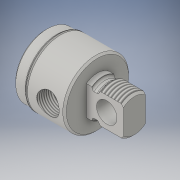
# Autodesk Inventor part: 09P0Y000_rear_head
Saved by Autodesk Inventor 2016 SP1 (Build 200210100, 210)
## iProperties
Category: PARTsolutions
Company: BIMBA
Created: 2017-03-09
Part Number: 09P0Y000_rear_head
Material: Generic
Catalog Web Link: www.cadenas.de
Description: Rear Head-Original Line - Standard Air Cylinders
Vendor: BIMBA
Document SubType Name: Standard Catalog Part
Designer: 589013
Manufacturer: BIMBA
Mass: 12.8763 g
Surface Area: 50.2035 cm^2
Volume: 12.8763 cm^3
Density: 1 g/cm^3
Appearance: PSOLRGB-211-211-211
PSOL_IDENT_0: {$CADENAS_DATA\23d-libs\bimba\bimba\bimba_imperial\bimba_full_line\original_line_cylinders\standard_
PSOL_IDENT_1: air_cylinders\rear_head.prj},231 {VTYP=3D},{NB=09P0Y000_rear_head},{LINA=09P0Y000_rear_head},{NN=Rea
PSOL_IDENT_2: r Head},{DATE=09.11.2016 07:55:11},{GEOMDATE=30.06.2014 06:34:00},{VERSION=},{LINEID=60},{LINESUBID=
PSOL_IDENT_3: -1},{WBVAR=MNT,ACTING,DER,Q,T1,T2,T3,T4,TRIM,Y,K,MB,CUSH,FBON}  {NB=09P0Y000_rear_head},{LINA=09P0Y0
PSOL_IDENT_4: 00_rear_head},{KT=DUMMY},{PN=09P0Y000},{BORE=1.06250},{BOREPN=09},{MNT=P},{MNTALG='' , 'Front Nose'
PSOL_IDENT_5: , 'P' , 'Rear Pivot' , 'S' , 'Built-in Valve S' , 'LS' , 'Built-in Valve LS' , 'DX' , 'Double End' ,
PSOL_IDENT_6: 'BR' , 'Rear Block' , 'BRT' , 'Rear Trunnion' , 'A' , 'Adjustable Stroke' , 'M' , 'Manual Valve'},{
PSOL_IDENT_7: ACTING=},{ACTINGALG= '' , 'Single Acting' , 'R' , 'Reverse/Double Acting' },{DER=},{DERALG= '' , 'St
PSOL_IDENT_8: andard' },{Q=},{T1=},{T2=},{T3=},{T4=},{TRIM=0},{Y=Y},{K=},{KALG= '', 'without K', 'K', 'with K' },{
PSOL_IDENT_9: MB=0},{A1=1.5000},{A1N=0.6250},{A1P=1.5000},{A1B=1.1250},{A1S=1.1250},{A2=0.25},{A2N=0.2500},{A3=0.0
PSOL_IDENT_10: 300},{D1=1.1110},{D1N=1.1155},{D1P=1.1110},{D1B=1.1410},{D2=1.0715},{C1=0.0300},{C2=0.0300},{NDM=0.4
PSOL_IDENT_11: 050},{TAB=NPT},{NDMDP=0.2730},{D3=0.3440},{A4=0.1880},{A5=0.8700},{D4=0.0000},{A6=0.0000},{A7=0.6250
PSOL_IDENT_12: },{A8=0.0000},{D5=0.0000},{D6=0.3750},{A9=0.7500},{NDM2=0.6250},{TAB2=UNF},{C11=0.0300},{C22=0.0000}
PSOL_IDENT_13: ,{C33=0.0000},{C44=0.0300},{A10=0.3725},{A11=0.0000},{NDM3=0.4050},{NDM3N=0.4050},{NDM3B=0.4050},{TA
PSOL_IDENT_14: B3=NPT},{TAB3N=NPT},{TAB3B=NPT},{A12=0.594},{A12N=0.5940},{A12B=0.6880},{A13=1.2190},{D7=0.2520},{D8=
PSOL_IDENT_15: 0.6225},{A14=0.0940},{A15=0.0855},{D9=0.5385},{R1=0.0350},{X1=0.0000},{X2=0.0000},{CX=0.0000},{CC=0.
PSOL_IDENT_16: 0000},{CON=1},{S1=1.2500},{DB=0.2500},{X1B=0.0000},{X2B=0.0000},{A8B=0.1250},{A9B=0.8800},{MODEL=1},
PSOL_IDENT_17: {NDM4=0.1900},{TAB4=UNF},{NDM4DP=0.3120},{BC=1.2500},{B1=0.7500},{B2=0.3800},{B3=0.5000},{ON=0},{ON2=
PSOL_IDENT_18: 1},{G1=0.3440},{G2=0.8120},{G3=0.6250},{G4=0.6245},{GD=0.2520},{G5=0.7180},{G6=0.3725},{RON=0},{H1=0
PSOL_IDENT_19: .0000},{H2=1.1300},{H3=0.1250},{H4=0.0000},{H5=0.0000},{H6=0.0000},{F=0.5000},{PNUT=0.9690},{CUSH=0}
PSOL_IDENT_20: ,{CC11=0.278},{CC111=0.2775},{CC22=0.4045},{CC33=0.2450},{CC44=0.5350},{CC55=0.7000},{CD1=0.2050},{C
PSOL_IDENT_21: D2=0.1360},{CD3=0.0775},{CNDM3=0.1900},{CTAB3=UNS},{OLEN=1.2190},{OD=0.3455},{STDIS=0.2500},{STDIS1=
PSOL_IDENT_22: 0.2500},{BUSHCON=D-3543},{BUSHL=0.3700},{FBON=0},{LCD=0.0000}
NN: Rear Head
NT: Original Line - Standard Air Cylinders
NB: 09P0Y000_rear_head
NBSYN: $PN._rear_head
LINA: 09P0Y000_rear_head
PN: 09P0Y000
BORE: 1.06250
BOREPN: 09
MNT: Rear Pivot
MNTALG: '' , 'Front Nose' , 'P' , 'Rear Pivot' , 'S' , 'Built-in Valve S' , 'LS' , 'Built-in Valve LS' , 'DX' , 'Double End' , 'BR' , 'Rear Block' , 'BRT' , 'Rear Trunnion' , 'A' , 'Adjustable Stroke' , 'M' , 'Manual Valve'
ACTING: Single Acting
DER: Standard
Q: Without Side Ported Rear Head
T1: without T1
T2: without T2
T3: without T3
T4: without T4
TRIM: 0
Y: with Pivot Bushing
K: without K
MB: 0
A1N: 0.6250
A1P: 1.5000
A1B: 1.1250
A1S: 1.1250
A2N: 0.2500
A3: 0.0300
D1N: 1.1155
D1P: 1.1110
D1B: 1.1410
D2: 1.0715
C1: 0.0300
C2: 0.0300
TAB: NPT
NDMDP: 0.2730
D3: 0.3440
A4: 0.1880
A5: 0.8700
D4: 0.0000
A6: 0.0000
A7: 0.6250
A8: 0.0000
D5: 0.0000
D6: 0.3750
A9: 0.7500
NDM2: 0.6250
TAB2: UNF
C11: 0.0300
C22: 0.0000
C33: 0.0000
C44: 0.0300
A10: 0.3725
A11: 0.0000
NDM3N: 0.4050
NDM3B: 0.4050
TAB3N: NPT
TAB3B: NPT
A12N: 0.5940
A12B: 0.6880
A13: 1.2190
D7: 0.2520
D8: 0.6225
A14: 0.0940
A15: 0.0855
D9: 0.5385
R1: 0.0350
X1: 0.0000
X2: 0.0000
CX: 0.0000
CC: 0.0000
S1: 1.2500
DB: 0.2500
X1B: 0.0000
X2B: 0.0000
A8B: 0.1250
A9B: 0.8800
NDM4: 0.1900
TAB4: UNF
NDM4DP: 0.3120
BC: 1.2500
B1: 0.7500
B2: 0.3800
B3: 0.5000
G1: 0.3440
G2: 0.8120
G3: 0.6250
G4: 0.6245
GD: 0.2520
G5: 0.7180
G6: 0.3725
H2: 1.1300
H3: 0.1250
F: 0.5000
CUSH: 0
CC111: 0.2775
CC22: 0.4045
CC33: 0.2450
CC44: 0.5350
CC55: 0.7000
CD1: 0.2050
CD2: 0.1360
CD3: 0.0775
CNDM3: 0.1900
CTAB3: UNS
OD: 0.3455
STDIS1: 0.2500
BUSHCON: D-3543
BUSHL: 0.3700
FBON: 0
LCD: 0.0000
SUPPLIER: BIMBA
ARTICLENO: 09P0Y000_rear_head
BOMINFO: 09P0Y000_rear_head
CREATOR: CADENAS GmbH
Title: 09P0Y000_rear_head
Author: Cadenas PARTsolutions
Comments: Original Line - Standard Air Cylinders
Autodesk Inventor part; units mm, degrees
ref_plane "YZ Plane" through (0, 0, 0) normal (1, 0, 0) x (0, 1, 0)
ref_plane "XZ Plane" through (0, 0, 0) normal (0, 1, 0) x (-1, 0, 0)
ref_plane "XY Plane" through (0, 0, 0) normal (0, 0, 1) x (1, 0, 0)
sketch "Sketch_18" plane through (0, 0, 0) normal (0, 0, 1) x (1, 0, 0)
  line L0 (22.225, 0) -> (0, 0)
  line L1 (0, 0) -> (0, 12.846)
  line L2 (0, 12.846) -> (0.762, 13.6081)
  line L3 (0.762, 13.6081) -> (4.826, 13.6081)
  line L4 (4.826, 13.6081) -> (5.588, 12.846)
  line L5 (5.588, 12.846) -> (6.35, 12.846)
  line L6 (6.35, 12.846) -> (6.35, 14.1097)
  line L7 (6.35, 14.1097) -> (21.463, 14.1097)
  line L8 (21.463, 14.1097) -> (22.225, 13.3477)
  line L9 (22.225, 13.3477) -> (22.225, 0)
  line L10 (22.225, 0) -> (0, 0)
  constraints: 22 end point
revolve "Revolution1" add sketch "Sketch_18" angle 360 about axis through (22.225, 0, 0) along (1, 0, 0)
sketch "Sketch_15" plane through (0, 0, 0) normal (0, 0, 1) x (1, 0, 0)
  line L0 (38.1, 0) -> (22.225, 0)
  line L1 (22.225, 0) -> (22.225, 7.9057)
  line L2 (22.225, 7.9057) -> (24.6126, 7.9057)
  line L3 (24.6126, 7.9057) -> (24.6126, 7.7279)
  arc A0 (24.6126, 7.7279) -> (25.5016, 6.839) centre (25.5016, 7.7279) ccw
  line L4 (25.5016, 6.839) -> (26.7843, 6.839)
  arc A1 (26.7843, 6.839) -> (27.383, 7.0708) centre (26.7843, 7.7279) ccw
  line L5 (27.383, 7.0708) -> (27.4129, 7.098)
  line L6 (27.4129, 7.098) -> (28.2524, 7.9375)
  line L7 (28.2524, 7.9375) -> (37.2605, 7.9375)
  line L8 (37.2605, 7.9375) -> (38.1, 7.098)
  line L9 (38.1, 7.098) -> (38.1, 0)
  line L10 (38.1, 0) -> (22.225, 0)
  constraints: 22 end point, 4 point on circle, 2 centre point
revolve "Revolution2" add sketch "Sketch_15" angle 360 about axis through (38.1, 0, 0) along (1, 0, 0)
thread "Thread1" size "5/8-18 UNF" class "2A" standard "ANSI Unified Screw Threads" full length
sketch "Sketch_9" plane through (38.1, 0, 0) normal (1, 0, 0) x (0, 0, -1)
  line L0 (-28.2194, -56.4388) -> (28.2194, -56.4388)
  line L1 (28.2194, -56.4388) -> (28.2194, 56.4388)
  line L2 (28.2194, 56.4388) -> (-28.2194, 56.4388)
  line L3 (-28.2194, 56.4388) -> (-28.2194, -56.4388)
  line L4 (-4.7307, -28.2194) -> (4.7307, -28.2194)
  line L5 (4.7307, -28.2194) -> (4.7307, 28.2194)
  line L6 (4.7307, 28.2194) -> (-4.7307, 28.2194)
  line L7 (-4.7307, 28.2194) -> (-4.7307, -28.2194)
  constraints: 16 end point
extrude "Extrusion1" cut sketch "Sketch_9" against normal blind 15.875
sketch "Sketch4" plane through (0, 0, 0) normal (-1, 0, 0) x (0, 0, 1)
  point P0 (0, 0)
hole "Hole1" at (0, 0, 0) direction (1, 0, 0) diameter 9.525 depth 20.955 tip angle 120
sketch "Sketch_68" plane through (0, 0, 0) normal (0, 0.9998477, 0.0174524) x (1, 0, 0)
  line L0 (15.0876, -14.1097) -> (15.0876, 0)
  line L1 (15.0876, 0) -> (19.7106, 0)
  line L2 (19.7106, 0) -> (19.7106, -7.1755)
  line L3 (19.7106, -7.1755) -> (19.9271, -14.1097)
  line L4 (19.9271, -14.1097) -> (15.0876, -14.1097)
  line L5 (15.0876, -14.1097) -> (15.0876, 0)
  constraints: 12 end point
revolve "Revolution3" cut sketch "Sketch_68" angle 360 about axis through (15.0876, -0.2462, 14.1076) along (0, -0.0174524, 0.9998477)
thread "Thread2" size "1/8" designation "1/8 - 27 NPT" standard "NPT" length 6.9376
sketch "Sketch_24" plane through (0, 0, 0) normal (0, 0, 1) x (1, 0, 0)
  line L0 (6.35, 0) -> (5.588, 0)
  line L1 (5.4861, 14.1097) -> (5.4861, 14.0255)
  line L2 (5.4861, 14.0255) -> (6.2275, 13.2842)
  arc A0 (6.2275, 13.1046) -> (6.2275, 13.2842) centre (6.1377, 13.1944) ccw
  line L3 (6.2275, 13.1046) -> (5.969, 12.846)
  line L4 (5.969, 12.846) -> (5.588, 12.846)
  line L5 (5.588, 12.846) -> (5.588, 12.5921)
  line L6 (5.588, 12.5921) -> (6.35, 12.5921)
  line L7 (6.35, 12.5921) -> (6.35, 13.449)
  line L8 (6.35, 13.449) -> (5.6893, 14.1097)
  line L9 (5.6893, 14.1097) -> (5.4861, 14.1097)
  constraints: 20 end point, 2 point on circle, 1 centre point
revolve "Revolution4" add sketch "Sketch_24" angle 360 about axis through (6.35, 0, 0) along (1, 0, 0)
sketch "Sketch_43" plane through (0, 0, 0) normal (0, 0, 1) x (1, 0, 0)
  circle A0 centre (30.9626, 0) radius 4.3879
  constraints: 1 centre point
extrude "Extrusion2" cut sketch "Sketch_43" along normal mid plane 14.1922
ref_plane "1_XY" through (24.6126, 0, 0) normal (1, 0, 0) x (0, 0, -1)
ref_plane "1_YZ" through (24.6126, 0, 0) normal (0, 0, -1) x (0, 1, 0)
ref_plane "1_ZX" through (24.6126, 0, 0) normal (0, 1, 0) x (1, 0, 0)
ref_plane "c1_XY" through (22.225, 7.9057, 0) normal (0, 0, 1) x (1, 0, 0)
ref_plane "c1_YZ" through (22.225, 7.9057, 0) normal (1, 0, 0) x (0, 1, 0)
ref_plane "c1_ZX" through (22.225, 7.9057, 0) normal (0, 1, 0) x (0, 0, 1)
ref_plane "c2_XY" through (22.225, -7.9057, 0) normal (0, 0, 1) x (1, 0, 0)
ref_plane "c2_YZ" through (22.225, -7.9057, 0) normal (1, 0, 0) x (0, 1, 0)
ref_plane "c2_ZX" through (22.225, -7.9057, 0) normal (0, 1, 0) x (0, 0, 1)
ref_plane "cc1_XY" through (22.225, 0, 0) normal (0, 0, 1) x (1, 0, 0)
ref_plane "cc1_YZ" through (22.225, 0, 0) normal (1, 0, 0) x (0, 1, 0)
ref_plane "cc1_ZX" through (22.225, 0, 0) normal (0, 1, 0) x (0, 0, 1)
ref_plane "cc2_XY" through (24.6126, 0, 0) normal (0, 0, 1) x (1, 0, 0)
ref_plane "cc2_YZ" through (24.6126, 0, 0) normal (1, 0, 0) x (0, 1, 0)
ref_plane "cc2_ZX" through (24.6126, 0, 0) normal (0, 1, 0) x (0, 0, 1)
ref_plane "lovra1_XY" through (33.3248, 0, 0) normal (1, 0, 0) x (0, 0, -1)
ref_plane "lovra1_YZ" through (33.3248, 0, 0) normal (0, 0, -1) x (0, 1, 0)
ref_plane "lovra1_ZX" through (33.3248, 0, 0) normal (0, 1, 0) x (1, 0, 0)
ref_plane "lovra2_XY" through (33.3248, 11.049, 0) normal (1, 0, 0) x (0, 0, -1)
ref_plane "lovra2_YZ" through (33.3248, 11.049, 0) normal (0, 0, -1) x (0, 1, 0)
ref_plane "lovra2_ZX" through (33.3248, 11.049, 0) normal (0, 1, 0) x (1, 0, 0)
ref_plane "lovra21_XY" through (0, 0, 5.2705) normal (1, 0, 0) x (0, 0, -1)
ref_plane "lovra21_YZ" through (0, 0, 5.2705) normal (0, 0, -1) x (0, 1, 0)
ref_plane "lovra21_ZX" through (0, 0, 5.2705) normal (0, 1, 0) x (1, 0, 0)
ref_plane "lovra22_XY" through (0, 0, -5.2705) normal (1, 0, 0) x (0, 0, -1)
ref_plane "lovra22_YZ" through (0, 0, -5.2705) normal (0, 0, -1) x (0, 1, 0)
ref_plane "lovra22_ZX" through (0, 0, -5.2705) normal (0, 1, 0) x (1, 0, 0)
ref_plane "lovra3_XY" through (33.3248, -11.049, 0) normal (1, 0, 0) x (0, 0, -1)
ref_plane "lovra3_YZ" through (33.3248, -11.049, 0) normal (0, 0, -1) x (0, 1, 0)
ref_plane "lovra3_ZX" through (33.3248, -11.049, 0) normal (0, 1, 0) x (1, 0, 0)
ref_plane "olen_XY" through (30.9626, 0, 0) normal (1, 0, 0) x (0, 0, -1)
ref_plane "olen_YZ" through (30.9626, 0, 0) normal (0, 0, -1) x (0, 1, 0)
ref_plane "olen_ZX" through (30.9626, 0, 0) normal (0, 1, 0) x (1, 0, 0)
ref_plane "p1_XY" through (38.1, 0, 4.7307) normal (1, 0, 0) x (0, 0, -1)
ref_plane "p1_YZ" through (38.1, 0, 4.7307) normal (0, 0, -1) x (0, 1, 0)
ref_plane "p1_ZX" through (38.1, 0, 4.7307) normal (0, 1, 0) x (1, 0, 0)
ref_plane "p2_XY" through (38.1, 0, -4.7307) normal (1, 0, 0) x (0, 0, -1)
ref_plane "p2_YZ" through (38.1, 0, -4.7307) normal (0, 0, -1) x (0, 1, 0)
ref_plane "p2_ZX" through (38.1, 0, -4.7307) normal (0, 1, 0) x (1, 0, 0)
ref_plane "port_XY" through (15.0876, 0, 0) normal (0, 0, 1) x (1, 0, 0)
ref_plane "port_YZ" through (15.0876, 0, 0) normal (1, 0, 0) x (0, 1, 0)
ref_plane "port_ZX" through (15.0876, 0, 0) normal (0, 1, 0) x (0, 0, 1)
ref_plane "port2_XY" through (38.1, 0, 0) normal (1, 0, 0) x (0, 0, -1)
ref_plane "port2_YZ" through (38.1, 0, 0) normal (0, 0, -1) x (0, 1, 0)
ref_plane "port2_ZX" through (38.1, 0, 0) normal (0, 1, 0) x (1, 0, 0)
ref_plane "thd1_XY" through (38.1, 0, 7.9375) normal (1, 0, 0) x (0, 0, -1)
ref_plane "thd1_YZ" through (38.1, 0, 7.9375) normal (0, 0, -1) x (0, 1, 0)
ref_plane "thd1_ZX" through (38.1, 0, 7.9375) normal (0, 1, 0) x (1, 0, 0)
ref_plane "thd2_XY" through (38.1, 0, -7.9375) normal (1, 0, 0) x (0, 0, -1)
ref_plane "thd2_YZ" through (38.1, 0, -7.9375) normal (0, 0, -1) x (0, 1, 0)
ref_plane "thd2_ZX" through (38.1, 0, -7.9375) normal (0, 1, 0) x (1, 0, 0)
ref_plane "to_mounting_bracket_XY" through (22.225, 0, 0) normal (1, 0, 0) x (0, 0, -1)
ref_plane "to_mounting_bracket_YZ" through (22.225, 0, 0) normal (0, 0, -1) x (0, 1, 0)
ref_plane "to_mounting_bracket_ZX" through (22.225, 0, 0) normal (0, 1, 0) x (1, 0, 0)
ref_plane "to_nut_XY" through (24.6126, 0, 0) normal (1, 0, 0) x (0, 0, -1)
ref_plane "to_nut_YZ" through (24.6126, 0, 0) normal (0, 0, -1) x (0, 1, 0)
ref_plane "to_nut_ZX" through (24.6126, 0, 0) normal (0, 1, 0) x (1, 0, 0)
ref_plane "to_pin_XY" through (30.9626, 0, 0) normal (0, 0, 1) x (1, 0, 0)
ref_plane "to_pin_YZ" through (30.9626, 0, 0) normal (1, 0, 0) x (0, 1, 0)
ref_plane "to_pin_ZX" through (30.9626, 0, 0) normal (0, 1, 0) x (0, 0, 1)
ref_plane "to_screw_XY" through (15.0876, 10.2743, -7.0612) normal (0, 1, 0) x (1, 0, 0)
ref_plane "to_screw_YZ" through (15.0876, 10.2743, -7.0612) normal (1, 0, 0) x (0, 0, -1)
ref_plane "to_screw_ZX" through (15.0876, 10.2743, -7.0612) normal (0, 0, -1) x (0, 1, 0)
ref_plane "to_tube_XY" through (5.588, 0, 0) normal (1, 0, 0) x (0, 0, -1)
ref_plane "to_tube_YZ" through (5.588, 0, 0) normal (0, 0, -1) x (0, 1, 0)
ref_plane "to_tube_ZX" through (5.588, 0, 0) normal (0, 1, 0) x (1, 0, 0)
body "Solid1"
